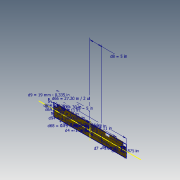
# Autodesk Inventor part: FLUGGER FRT FASCIA PANEL
Saved by Autodesk Inventor 2020.3 (Build 243373000, 373)
## iProperties
RuleStatus: InUse
AfterDocSave0: file://Part Number Cleaner
Created: 2019-10-25
Material: ACRYLIC, BLACK
Vendor: HHMI: JRC - ID&F
Document SubType Name: Modeling
Designer: arnoldj
Density: 1 g/cm^3
Appearance: Gold
DESIGN DEPARTMENT: HHMI: JRC - ID&F
ALTERED ITEM PART NUMBER: N/A
ALTERED ITEM VENDOR: N/A
ALTERED ITEM DESCRIPTION: N/A
Author: arnoldj
Revision Number: 0
Autodesk Inventor part; units mm, degrees
ref_plane "YZ Plane" through (0, 0, 0) normal (1, 0, 0) x (0, 1, 0)
ref_plane "XZ Plane" through (0, 0, 0) normal (0, 1, 0) x (-1, 0, 0)
ref_plane "XY Plane" through (0, 0, 0) normal (0, 0, 1) x (1, 0, 0)
sketch "Sketch1" plane through (0, 0, 0) normal (0, 0, 1) x (1, 0, 0)
  line L0 (0, 88.9) -> (0, -88.9) projected
  line L1 (-533.4, 0) -> (533.4, 0) projected
  line L2 (381, -63.5) -> (-381, -63.5)
  line L3 (-381, -63.5) -> (-381, 63.5)
  line L4 (-381, 63.5) -> (381, 63.5)
  line L5 (381, 63.5) -> (381, -63.5)
  line L6 (381, -63.5) -> (-381, 63.5) construction
  line L7 (-381, -63.5) -> (381, 63.5) construction
  line L8 (-170.942, -37.592) -> (-127, -37.592) construction
  line L9 (-127, -37.592) -> (-127, -63.5) construction
  line L10 (-127, -63.5) -> (-170.942, -63.5) construction
  line L11 (-170.942, -63.5) -> (-170.942, -37.592) construction
  line L12 (127, -37.592) -> (170.942, -37.592) construction
  line L13 (170.942, -37.592) -> (170.942, -63.5) construction
  line L14 (170.942, -63.5) -> (127, -63.5) construction
  line L15 (127, -63.5) -> (127, -37.592) construction
  line L16 (-381, 31.75) -> (-345.44, 31.75)
  line L17 (-345.44, 31.75) -> (-345.44, 63.5)
  line L18 (345.44, 63.5) -> (345.44, 31.75)
  line L19 (345.44, 31.75) -> (381, 31.75)
  line L20 (368.3, -44.45) -> (-368.3, -44.45) construction
  line L21 (-368.3, -44.45) -> (-368.3, 12.7) construction
  line L22 (-368.3, 12.7) -> (368.3, 12.7) construction
  line L23 (368.3, 12.7) -> (368.3, -44.45) construction
  line L24 (368.3, -44.45) -> (-368.3, 12.7) construction
  line L25 (-368.3, -44.45) -> (368.3, 12.7) construction
  line L26 (328.6125, -23.8125) -> (357.1875, -23.8125)
  line L27 (357.1875, -23.8125) -> (357.1875, 23.8125)
  line L28 (357.1875, 23.8125) -> (328.6125, 23.8125)
  line L29 (328.6125, 23.8125) -> (328.6125, -23.8125)
  line L30 (328.6125, -23.8125) -> (357.1875, 23.8125) construction
  line L31 (357.1875, -23.8125) -> (328.6125, 23.8125) construction
  line L32 (-42.8625, -23.8125) -> (-14.2875, -23.8125)
  line L33 (-14.2875, -23.8125) -> (-14.2875, 23.8125)
  line L34 (-14.2875, 23.8125) -> (-42.8625, 23.8125)
  line L35 (-42.8625, 23.8125) -> (-42.8625, -23.8125)
  line L36 (-42.8625, -23.8125) -> (-14.2875, 23.8125) construction
  line L37 (-14.2875, -23.8125) -> (-42.8625, 23.8125) construction
  point P0 (0, 0)
  point P1 (-159.004, -63.5)
  point P2 (138.938, -63.5)
  point P3 (-279.4, 53.009)
  point P4 (279.4, 53.009)
  point P5 (-5.08, 53.009)
  point P6 (0, -15.875)
  point P7 (342.9, 0)
  point P8 (-28.575, 0)
  point P9 (-368.3, -15.875)
  point P10 (368.3, -15.875)
  dimension "d0" = 762
  dimension "d1" = 127
  dimension "d2" = 43.942
  dimension "d3" = 25.908
  dimension "d4" = 32.004
  dimension "d5" = 127
  dimension "d7" = 32.004
  dimension "d8" = 127
  dimension "d9" = 10.491
  dimension "d65" = 31.75
  dimension "d66" = 345.44
  dimension "d67" = 736.6
  dimension "d68" = 19.05
  dimension "d69" = 19.05
  dimension "d84" = 279.4
  dimension "d85" = 279.4
  dimension "d86" = 5.08
  dimension "d87" = 28.575
  dimension "d88" = 47.625
  dimension "d89" = 0
  dimension "d90" = 28.575
  dimension "d91" = 342.9
  dimension "d94" = 101.092
  constraints: 72 end point, 12 parallel, 10 midpoint, 10 point on line, 8 coincident, 8 perpendicular, 7 horizontal, 5 equal length, 2 horizontal alignment, 1 vertical
  measures "d0" distance of L3.end L4.end
  measures "d1" distance of L2.end L3.end
  measures "d2" distance of L8.start L8.end
  measures "d3" distance of L10.end L8.start
  measures "d4" distance from line of L9 point (-159.004, -63.5)
  measures "d5" distance between parallel lines of L0 L9
  measures "d7" distance from line of L13 point (138.938, -63.5)
  measures "d8" distance between parallel lines of L0 L15
  measures "d9" distance from line of point (-279.4, 53.009) L4
  measures "d65" distance of L16.end L17.end
  measures "d66" distance between parallel lines of L0 L17
  measures "d67" distance of L21.end L22.end
  measures "d68" distance between parallel lines of L20 L2
  measures "d69" distance between parallel lines of L22 L16
  measures "d84" distance from line of L0 point (-279.4, 53.009)
  measures "d85" distance from line of point (279.4, 53.009) L0
  measures "d86" distance from line of L0 point (-5.08, 53.009)
  measures "d87" distance of L33.end L34.end
  measures "d88" distance of L26.end L27.end
  measures "d89" distance from line of point (-28.575, 0) L1
  measures "d90" distance from line of L0 point (-28.575, 0)
  measures "d91" distance from line of point (342.9, 0) L0
  measures "d94" distance from line of point (-170.942, -37.592) L4
extrude "Extrusion1" add sketch "Sketch1" against normal blind 5.842 contours L4 L18 L19 L5 L1 L27 L28 L29 L0 | L0 L1 L33 L34 L35 L3 L16 L17 L4 | L1 L29 L26 L27 L5 L2 L0 | L0 L2 L3 L1 L35 L32 L33 | L33 L32 L35 L1 | L1 L35 L34 L33 | L29 L28 L27 L1 | L1 L27 L26 L29
hole "Hole2" at (-279.4, 53.009, 0) at (279.4, 53.009, 0) at (-5.08, 53.009, 0) direction (0, 0, -1) diameter 6.731 end through all
fillet "Fillet1" radius 9.525 2 edges at (381, -63.5, -2.921) (-381, -63.5, -2.921)
hole "Hole5" at (-368.3, -15.875, 0) at (368.3, -15.875, 0) direction (0, 0, -1) diameter 7.0104 end through all clearance for "Socket Head Cap Screw" size "M6" standard "Ansi Metric M Profile"
fillet "Fillet2" radius 1.905 6 edges at (-381, 31.75, -2.921) (-345.44, 31.75, -2.921) (-345.44, 63.5, -2.921) (345.44, 63.5, -2.921) (381, 31.75, -2.921) (345.44, 31.75, -2.921)
sketch "Sketch4" plane through (0, 0, 0) normal (0, 0, 1) x (1, 0, 0)
  line L0 (343.535, 63.5) -> (-343.535, 63.5) projected
  line L1 (208.5594, 31.75) -> (160.2994, 31.75)
  line L2 (160.2994, 31.75) -> (160.2994, 63.5)
  line L3 (160.2994, 63.5) -> (208.5594, 63.5)
  line L4 (208.5594, 63.5) -> (208.5594, 31.75)
  line L5 (208.5594, 31.75) -> (160.2994, 63.5) construction
  line L6 (160.2994, 31.75) -> (208.5594, 63.5) construction
  line L7 (0, 88.9) -> (0, -88.9) projected
  point P0 (0, 0)
  point P1 (184.4294, 47.625)
  point P2 (208.5594, 63.5)
  dimension "d78" = 48.26
  dimension "d80" = 31.75
  dimension "d83" = 184.4294
  constraints: 12 end point, 2 midpoint, 2 parallel, 1 horizontal, 1 perpendicular, 1 point on line
  measures "d78" distance of L1.start L1.end
  measures "d80" distance of L1.end L2.end
  measures "d83" distance from line of point (184.429, 47.625) L7
extrude "Extrusion2" cut sketch "Sketch4" against normal through all
fillet "Fillet3" radius 1.905 4 edges at (160.2994, 63.5, -2.921) (160.2994, 31.75, -2.921) (208.5594, 31.75, -2.921) (208.5594, 63.5, -2.921)
sketch "Sketch5" plane through (0, 0, 0) normal (0, 0, 1) x (1, 0, 0)
  line L0 (371.475, -63.5) -> (-371.475, -63.5) projected
  line L1 (0, 88.9) -> (0, -88.9) projected
  line L2 (330.2, -50.8) -> (-330.2, -50.8) construction
  line L3 (-371.475, -63.5) -> (371.475, -63.5) construction
  point P0 (0, 0)
  point P1 (0, -50.8)
  point P2 (165.1, -50.8)
  point P3 (-165.1, -50.8)
  dimension "d108" = 330.2
  dimension "d109" = 330.2
  dimension "d110" = 12.7
  dimension "d118" = 165.1
  dimension "d119" = 165.1
  constraints: 3 point on line, 2 coincident, 2 end point, 1 midpoint, 1 parallel
  measures "d108" distance from line of L1 point (-330.2, -50.8)
  measures "d109" distance from line of L1 point (330.2, -50.8)
  measures "d110" distance between parallel lines of L2 L0
  measures "d118" distance of point (330.2, -50.8) point (165.1, -50.8)
  measures "d119" distance of point (-330.2, -50.8) point (-165.1, -50.8)
hole "Hole6" at (330.2, -50.8, 0) at (0, -50.8, 0) at (-330.2, -50.8, 0) at (165.1, -50.8, 0) at (-165.1, -50.8, 0) direction (0, 0, -1) diameter 3.1242 end through all
pattern_linear "Rectangular Pattern2" count 2 spacing 25.4 along (0, 1, 0) of "Hole6"
equation "\"d118\" = 0.5 * d109"
equation "\"d119\" = 0.5 * d109"
body "Solid1"
